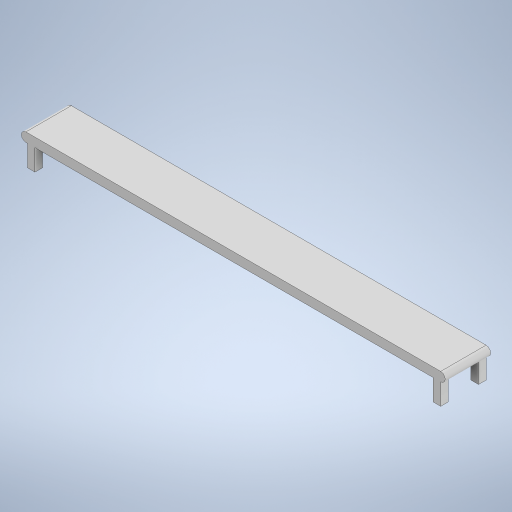
# Autodesk Inventor part: SoporteBanda
Saved by Autodesk Inventor 2024 (Build 280153000, 153)
## iProperties
Created: 2024-06-27
Part Number: SoporteBanda
Material: Genérico
Document SubType Name: Modeling
Designer: USER
Density: 1 g/cm^3
Appearance: Valor por defecto
Author: USER
Autodesk Inventor part; units mm, degrees
ref_plane "YZ Plane" through (0, 0, 0) normal (1, 0, 0) x (0, 1, 0)
ref_plane "XZ Plane" through (0, 0, 0) normal (0, 1, 0) x (-1, 0, 0)
ref_plane "XY Plane" through (0, 0, 0) normal (0, 0, 1) x (1, 0, 0)
sketch "Boceto1" plane through (0, 0, 0) normal (0, 1, 0) x (-1, 0, 0)
  line L0 (7000, -750) -> (-7000, -750)
  line L1 (-7000, -750) -> (-7000, 750)
  line L2 (-7000, 750) -> (7000, 750)
  line L3 (7000, 750) -> (7000, -750)
  line L4 (7000, -750) -> (-7000, 750) construction
  line L5 (-7000, -750) -> (7000, 750) construction
  point P0 (0, 0)
  dimension "d0" = 14000
  dimension "d1" = 1500
  constraints: 12 end point, 2 midpoint, 2 parallel, 1 horizontal, 1 perpendicular
  measures "d0" distance of L1.end L2.end
  measures "d1" distance between parallel lines of L0 L2
extrude "Extrusión1" add sketch "Boceto1" along normal blind 300
sketch "Boceto2" plane through (-7000, 0, 750) normal (0, 0, 1) x (1, 0, 0)
  line L0 (14000, 0) -> (14000, 300) projected
  line L1 (0, 300) -> (14000, 300) projected
  line L2 (0, 0) -> (14000, 0) projected
  line L3 (0, 0) -> (0, 300) projected
  circle A0 centre (13850, 150) radius 150
  circle A1 centre (150, 150) radius 150
  line L4 (13850, 300) -> (14000, 300)
  line L5 (14000, 0) -> (13850, 0)
  line L6 (150, 0) -> (0, 0)
  line L7 (0, 300) -> (150, 300)
  line L8 (0, 0) -> (0, 300)
  line L9 (14000, 0) -> (14000, 300)
  point P0 (7000, 0)
  point P1 (14000, 150)
  point P2 (0, 150)
  constraints: 12 end point, 8 tangent, 4 point on circle, 4 point on line, 3 collinear, 2 centre point, 1 parallel
extrude "Extrusión2" cut sketch "Boceto2" against normal through all contours L2 A0 L0 | A0 L1 L0 | L2 L3 A1 | A1 L3 L1
sketch "Boceto3" plane through (0, 0, 0) normal (0, -1, 0) x (1, 0, 0)
  line L0 (-6850, 750) -> (6850, 750) projected
  line L1 (6850, -750) -> (6850, 750) projected
  line L2 (6850, -750) -> (-6850, -750) projected
  line L3 (-6850, -750) -> (-6850, 750) projected
  line L4 (6850, 750) -> (6850, 500)
  line L5 (6850, 500) -> (6600, 500)
  line L6 (6600, 500) -> (6600, 750)
  line L7 (6600, 750) -> (6850, 750)
  line L8 (6850, -500) -> (6850, -750)
  line L9 (6850, -750) -> (6600, -750)
  line L10 (6600, -750) -> (6600, -500)
  line L11 (6600, -500) -> (6850, -500)
  line L12 (-6550, 750) -> (-6550, 500)
  line L13 (-6550, 500) -> (-6800, 500)
  line L14 (-6800, 500) -> (-6800, 750)
  line L15 (-6800, 750) -> (-6550, 750)
  line L16 (-6550, -500) -> (-6550, -750)
  line L17 (-6550, -750) -> (-6800, -750)
  line L18 (-6800, -750) -> (-6800, -500)
  line L19 (-6800, -500) -> (-6550, -500)
  point P0 (0, 0)
  point P1 (6600, 750)
  point P2 (6600, -750)
  point P3 (-6800, 750)
  point P4 (-6800, -750)
  point P5 (-6550, -750)
  dimension "d6" = 250
  dimension "d7" = 250
  dimension "d10" = 1250
  dimension "d13" = 13400
  constraints: 32 end point, 2 parallel, 1 horizontal, 1 perpendicular, 1 point on line, 1 vertical, 24 other
  measures "d6" distance of L0.end L4.end
  measures "d7" distance of L4.end L5.end
  measures "d10" distance of L4.end L8.end
  measures "d13" distance of L4.end L12.end
extrude "Extrusión3" add sketch "Boceto3" along normal blind 700 contours L0 L12 L13 L14 | L18 L19 L16 L2 | L0 L1 L5 L6 | L10 L11 L1 L2
equation "\"d0\" = L"
equation "\"L\" = 14000"
